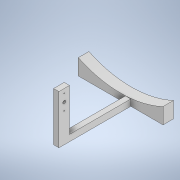
# Autodesk Inventor part: tete_statique
Saved by Autodesk Inventor 2020 (Build 240168000, 168)
## iProperties
Created: 2019-12-28
Part Number: tete_statique
Material: Générique
Document SubType Name: Modeling
Designer: bapti
Density: 1 g/cm^3
Appearance: Par défaut
Author: bapti
Autodesk Inventor part; units mm, degrees
ref_plane "YZ Plane" through (0, 0, 0) normal (1, 0, 0) x (0, 1, 0)
ref_plane "XZ Plane" through (0, 0, 0) normal (0, 1, 0) x (-1, 0, 0)
ref_plane "XY Plane" through (0, 0, 0) normal (0, 0, 1) x (1, 0, 0)
sketch "Esquisse1" plane through (0, 0, 0) normal (0, 0, 1) x (1, 0, 0)
  line L0 (0, 0) -> (0, 15)
  line L1 (0, 0) -> (80, 0)
  line L2 (80, 0) -> (80, 15)
  arc A0 (0, 15) -> (80, 15) centre (40, 99.3889) ccw
  line L3 (0, 6) -> (80, 6) construction
  line L4 (40, 0) -> (40, 6) construction
  dimension "d0" = 15
  dimension "d1" = 80
  dimension "d28" = 6
  constraints: 10 end point, 2 midpoint, 2 perpendicular, 2 point on circle, 2 point on line, 1 centre point, 1 horizontal, 1 parallel, 1 tangent, 1 vertical
  measures "d0" distance of L0.start L0.end
  measures "d1" distance of L0.start L1.end
  measures "d28" distance of L4.start L4.end
extrude "Extrusion1" add sketch "Esquisse1" along normal blind 10
sketch "Esquisse2" plane through (0, 0, 10) normal (0, 0, 1) x (1, 0, 0)
  line L0 (0, 0) -> (80, 0) projected
  line L1 (44.6, 0) -> (49.6, 0)
  line L2 (49.6, 0) -> (49.6, 6)
  line L3 (49.6, 6) -> (44.6, 6)
  line L4 (44.6, 6) -> (44.6, 0)
  line L5 (0, 15) -> (0, 0) projected
  line L6 (0, 6) -> (80, 6) construction
  line L7 (80, 0) -> (80, 15) projected
  arc A0 (0, 15) -> (80, 15) centre (40, 99.3889) ccw projected
  line L8 (40, 0) -> (40, 6) construction
  dimension "d6" = 5
  dimension "d9" = 80
  dimension "d11" = 6
  dimension "d27" = 4.6
  constraints: 12 end point, 3 point on line, 2 horizontal, 2 parallel, 1 midpoint, 1 perpendicular, 1 point on circle, 1 tangent
  measures "d6" distance of L2.end L3.end
  measures "d9" distance of L0.start L0.end
  measures "d11" distance of L3.end L1.start
  measures "d27" distance between parallel lines of L8 L4
extrude "Extrusion2" add sketch "Esquisse2" along normal blind 67.9 contours L4 L3 L2 L0
sketch "Esquisse6" plane through (44.6, 6, 10) normal (0, 1, 0) x (1, 0, 0)
  line L0 (5, 0) -> (5, -67.9) projected
  line L1 (0, 0) -> (0, -67.9) projected
  line L2 (5, -67.9) -> (0, -67.9)
  line L3 (0, -67.9) -> (0, -57.9)
  line L4 (0, -57.9) -> (5, -57.9)
  line L5 (5, -57.9) -> (5, -67.9)
  point P0 (-44.6, 10)
  point P1 (5, -57.9)
  dimension "d29" = 10
  constraints: 8 end point, 2 parallel, 1 horizontal, 1 perpendicular, 1 point on line
  measures "d29" distance of L1.end L3.end
extrude "Extrusion5" add sketch "Esquisse6" along normal blind 40
sketch "Esquisse7" plane through (44.6, 0, 10) normal (-1, 0, 0) x (0, 0, 1)
  circle A0 centre (62.9, 42) radius 0.5
  circle A1 centre (62.9, 27.8) radius 0.5
  line L0 (67.9, 46) -> (57.9, 46) construction
  line L1 (62.9, 46) -> (62.9, 0) construction
  line L2 (0, 0) -> (67.9, 0) construction
  circle A2 centre (62.9, 34.9) radius 3.3
  circle A3 centre (62.9, 34.9) radius 2.6
  circle A4 centre (62.9, 34.9) radius 1.4
  point P0 (-10, 0)
  dimension "d32" = 1
  dimension "d33" = 1
  dimension "d34" = 14.2
  dimension "d35" = 4
  dimension "d36" = 6.6
  dimension "d37" = 0.7
  dimension "d38" = 2.8
  dimension "d39" = 7.1
  constraints: 5 centre point, 4 point on line, 2 coincident, 2 end point, 1 midpoint, 1 vertical
  measures "d32" diameter of A0
  measures "d33" diameter of A1
  measures "d34" distance of A1.centre A0.centre
  measures "d35" distance from line of A0.centre L0
  measures "d36" diameter of A2
  measures "d37" radial gap between concentric circles of A2 A3
  measures "d38" diameter of A4
  measures "d39" distance of A2.centre A0.centre
extrude "Extrusion6" cut sketch "Esquisse7" against normal up to surface (5 mm away) contours A0 | A1 | A4
extrude "Extrusion7" cut sketch "Esquisse7" against normal blind 1.2 contours A2
equation "\"d33\" = d32"
equation "\"d39\" = 0.5 * d34"
